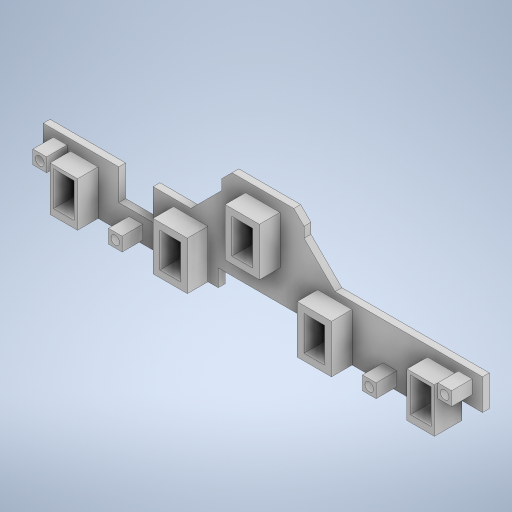
# Autodesk Inventor part: Infravermelhos_revisto_2
Saved by Autodesk Inventor 2024 (Build 280153000, 153)
## iProperties
Created: 2023-04-03
Part Number: Infravermelhos_revisto_2
Material: Generic
Document SubType Name: Modeling
Designer: guilh
Density: 1 g/cm^3
Appearance: Default
Author: guilh
Autodesk Inventor part; units mm, degrees
ref_plane "YZ Plane" through (0, 0, 0) normal (1, 0, 0) x (0, 1, 0)
ref_plane "XZ Plane" through (0, 0, 0) normal (0, 1, 0) x (-1, 0, 0)
ref_plane "XY Plane" through (0, 0, 0) normal (0, 0, 1) x (1, 0, 0)
sketch "Sketch1" plane through (0, 0, 0) normal (0, 0, 1) x (1, 0, 0)
  line L0 (-64, 31) -> (-73, 31)
  line L1 (-76, 28) -> (-76, 25)
  line L2 (-85, 16) -> (-76, 25)
  line L3 (-76, 28) -> (-73, 31)
  line L4 (-64, 31) -> (-55, 31)
  line L5 (-52, 28) -> (-52, 25)
  line L6 (-43, 16) -> (-52, 25)
  line L7 (-52, 28) -> (-55, 31)
  line L8 (-43, 16) -> (0, 16)
  line L9 (-77, 0) -> (-77, 5)
  line L10 (-77, 5) -> (-51, 5)
  line L11 (-51, 5) -> (-51, 0)
  line L12 (-106, 16) -> (-106, 7)
  line L13 (-106, 7) -> (-96, 7)
  line L14 (-96, 7) -> (-96, 16)
  line L15 (-128, 16) -> (-106, 16)
  line L16 (-96, 16) -> (-85, 16)
  line L17 (-120, 0) -> (-120, 7)
  line L18 (-120, 7) -> (-128, 7)
  line L19 (-120, 0) -> (-77, 0)
  line L20 (-128, 16) -> (-128, 7)
  line L21 (-8, 0) -> (-8, 7)
  line L22 (-8, 7) -> (0, 7)
  line L23 (-51, 0) -> (-8, 0)
  line L24 (0, 7) -> (0, 16)
  point P0 (0, 0)
  dimension "d0" = 128
  dimension "d6" = 3
  dimension "d67" = 5
  dimension "d71" = 22
  dimension "d74" = 9
  dimension "d75" = 10
  dimension "d93" = 7
  dimension "d94" = 8
  dimension "d95" = 7
  constraints: 50 end point, 6 horizontal, 3 perpendicular, 2 vertical
  measures "d0" distance of L15.start L8.end
  measures "d6" distance of L1.start L1.end
  measures "d67" distance of L9.start L9.end
  measures "d71" distance of L15.start L12.start
  measures "d74" distance of L12.start L12.end
  measures "d75" distance of L12.end L13.end
  measures "d93" distance of L17.start L17.end
  measures "d94" distance of point (0, 0) L21.start
  measures "d95" distance of L21.start L21.end
extrude "Extrusion1" add sketch "Sketch1" against normal blind 2
sketch "Sketch2" plane through (0, 0, 0) normal (0, 0, 1) x (1, 0, 0)
  line L0 (-119, 2) -> (-113, 2)
  line L1 (-113, 2) -> (-113, 12)
  line L2 (-113, 12) -> (-119, 12)
  line L3 (-119, 12) -> (-119, 2)
  line L4 (-121, 10) -> (-125, 10)
  line L5 (-125, 10) -> (-125, 14)
  line L6 (-125, 14) -> (-121, 14)
  line L7 (-121, 14) -> (-121, 10)
  line L8 (-88, 2) -> (-82, 2)
  line L9 (-82, 2) -> (-82, 12)
  line L10 (-82, 12) -> (-88, 12)
  line L11 (-88, 12) -> (-88, 2)
  line L12 (-90, 0) -> (-80, 0)
  line L13 (-80, 0) -> (-80, 14)
  line L14 (-80, 14) -> (-90, 14)
  line L15 (-90, 14) -> (-90, 0)
  line L16 (-99, 1) -> (-103, 1)
  line L17 (-103, 1) -> (-103, 5)
  line L18 (-103, 5) -> (-99, 5)
  line L19 (-99, 5) -> (-99, 1)
  line L20 (-61, 26) -> (-67, 26)
  line L21 (-67, 26) -> (-67, 16)
  line L22 (-67, 16) -> (-61, 16)
  line L23 (-61, 16) -> (-61, 26)
  line L24 (-59, 14) -> (-69, 14)
  line L25 (-69, 14) -> (-69, 28)
  line L26 (-69, 28) -> (-59, 28)
  line L27 (-59, 28) -> (-59, 14)
  line L28 (-9, 2) -> (-15, 2)
  line L29 (-15, 2) -> (-15, 12)
  line L30 (-15, 12) -> (-9, 12)
  line L31 (-9, 12) -> (-9, 2)
  line L32 (-7, 10) -> (-3, 10)
  line L33 (-3, 10) -> (-3, 14)
  line L34 (-3, 14) -> (-7, 14)
  line L35 (-7, 14) -> (-7, 10)
  line L36 (-40, 2) -> (-46, 2)
  line L37 (-46, 2) -> (-46, 12)
  line L38 (-46, 12) -> (-40, 12)
  line L39 (-40, 12) -> (-40, 2)
  line L40 (-38, 0) -> (-48, 0)
  line L41 (-48, 0) -> (-48, 14)
  line L42 (-48, 14) -> (-38, 14)
  line L43 (-38, 14) -> (-38, 0)
  line L44 (-29, 1) -> (-25, 1)
  line L45 (-25, 1) -> (-25, 5)
  line L46 (-25, 5) -> (-29, 5)
  line L47 (-29, 5) -> (-29, 1)
  line L48 (-112, 13) -> (-120, 13)
  line L49 (-8, 13) -> (-16, 13)
  line L50 (-120, 13) -> (-120, 0)
  line L51 (-112, 13) -> (-112, 0)
  line L52 (-16, 13) -> (-16, 0)
  line L53 (-8, 13) -> (-8, 0)
  circle A0 centre (-123, 12) radius 1.25
  circle A1 centre (-101, 3) radius 1.25
  circle A2 centre (-27, 3) radius 1.25
  circle A3 centre (-5, 12) radius 1.25
  line L54 (-120, 0) -> (-112, 0)
  line L55 (-16, 0) -> (-8, 0)
  dimension "d12" = 6
  dimension "d13" = 10
  dimension "d21" = 6
  dimension "d22" = 10
  dimension "d23" = 2
  dimension "d29" = 6
  dimension "d30" = 10
  dimension "d31" = 2
  dimension "d48" = 1
  dimension "d49" = 2.5
  dimension "d50" = 2.5
  dimension "d51" = 2.5
  dimension "d52" = 2.5
  dimension "d69" = 13
  constraints: 112 end point, 14 parallel, 7 perpendicular, 6 horizontal, 4 centre point, 1 vertical, 6 other
  measures "d12" distance of L2.end L1.end
  measures "d13" distance of L1.end L0.end
  measures "d21" distance of L10.end L9.end
  measures "d22" distance of L9.end L8.end
  measures "d23" distance between parallel lines of L11 L15
  measures "d29" distance of L22.end L21.end
  measures "d30" distance of L21.end L20.end
  measures "d31" distance between parallel lines of L22 L24
  measures "d48" distance between parallel lines of L30 L49
  measures "d49" diameter of A0
  measures "d50" diameter of A1
  measures "d51" diameter of A2
  measures "d52" diameter of A3
  measures "d69" distance of L51.end L48.start
sketch "Sketch10" plane through (0, 0, 0) normal (0, 0, 1) x (1, 0, 0)
  line L0 (-119, 2) -> (-113, 2)
  line L1 (-113, 2) -> (-113, 12)
  line L2 (-113, 12) -> (-119, 12)
  line L3 (-119, 12) -> (-119, 2)
  line L4 (-121, 10) -> (-125, 10)
  line L5 (-125, 10) -> (-125, 14)
  line L6 (-125, 14) -> (-121, 14)
  line L7 (-121, 14) -> (-121, 10)
  line L8 (-88, 2) -> (-82, 2)
  line L9 (-82, 2) -> (-82, 12)
  line L10 (-82, 12) -> (-88, 12)
  line L11 (-88, 12) -> (-88, 2)
  line L12 (-90, 0) -> (-80, 0)
  line L13 (-80, 0) -> (-80, 14)
  line L14 (-80, 14) -> (-90, 14)
  line L15 (-90, 14) -> (-90, 0)
  line L16 (-99, 1) -> (-103, 1)
  line L17 (-103, 1) -> (-103, 5)
  line L18 (-103, 5) -> (-99, 5)
  line L19 (-99, 5) -> (-99, 1)
  line L20 (-61, 26) -> (-67, 26)
  line L21 (-67, 26) -> (-67, 16)
  line L22 (-67, 16) -> (-61, 16)
  line L23 (-61, 16) -> (-61, 26)
  line L24 (-59, 14) -> (-69, 14)
  line L25 (-69, 14) -> (-69, 28)
  line L26 (-69, 28) -> (-59, 28)
  line L27 (-59, 28) -> (-59, 14)
  line L28 (-25, 1) -> (-25, 5)
  line L29 (-9, 2) -> (-15, 2)
  line L30 (-15, 2) -> (-15, 12)
  line L31 (-15, 12) -> (-9, 12)
  line L32 (-9, 12) -> (-9, 2)
  line L33 (-7, 14) -> (-7, 10)
  line L34 (-7, 10) -> (-3, 10)
  line L35 (-3, 10) -> (-3, 14)
  line L36 (-3, 14) -> (-7, 14)
  line L37 (-29, 1) -> (-25, 1)
  line L38 (-25, 5) -> (-29, 5)
  line L39 (-29, 5) -> (-29, 1)
  line L40 (-38, 14) -> (-38, 0)
  line L41 (-40, 12) -> (-40, 2)
  line L42 (-40, 2) -> (-46, 2)
  line L43 (-46, 12) -> (-40, 12)
  line L44 (-46, 2) -> (-46, 12)
  line L45 (-48, 14) -> (-38, 14)
  line L46 (-48, 0) -> (-48, 14)
  line L47 (-38, 0) -> (-48, 0)
  line L48 (-112, 13) -> (-120, 13)
  line L49 (-8, 13) -> (-16, 13)
  circle A0 centre (-123, 12) radius 1.25
  circle A1 centre (-101, 3) radius 1.25
  circle A2 centre (-27, 3) radius 1.25
  circle A3 centre (-5, 12) radius 1.25
  line L50 (-120, 13) -> (-120, 0)
  line L51 (-112, 13) -> (-112, 0)
  line L52 (-112, 0) -> (-120, 0)
  line L53 (-16, 13) -> (-16, 0)
  line L54 (-16, 0) -> (-8, 0)
  line L55 (-8, 13) -> (-8, 0)
  point P0 (-100.5385, 17.107)
  point P1 (-110.5385, 3.107)
  point P2 (-100.5385, 3.107)
  point P3 (-141.5385, 3.107)
  point P4 (-131.5385, 3.107)
  point P5 (-183.5385, 3.107)
  point P6 (-173.5385, 3.107)
  point P7 (-214.5385, 3.107)
  point P8 (-204.5385, 3.107)
  point P9 (-214.5385, 17.107)
  point P10 (0, 16)
  point P11 (0, 0)
  dimension "d53" = 6
  dimension "d54" = 10
  dimension "d55" = 6
  dimension "d56" = 10
  dimension "d57" = 2
  dimension "d58" = 6
  dimension "d59" = 10
  dimension "d60" = 2
  dimension "d61" = 1
  dimension "d62" = 2.5
  dimension "d63" = 2.5
  dimension "d64" = 2.5
  dimension "d65" = 2.5
  constraints: 112 end point, 14 parallel, 9 perpendicular, 5 horizontal, 4 centre point, 3 vertical, 6 other
  measures "d53" distance of L2.end L2.start
  measures "d54" distance of L2.start L0.end
  measures "d55" distance of L11.start L9.end
  measures "d56" distance of L9.end L8.end
  measures "d57" distance between parallel lines of L11 L15
  measures "d58" distance of L22.end L21.end
  measures "d59" distance of L21.end L21.start
  measures "d60" distance between parallel lines of L22 L24
  measures "d61" distance between parallel lines of L31 L49
  measures "d62" diameter of A0
  measures "d63" diameter of A1
  measures "d64" diameter of A2
  measures "d65" diameter of A3
extrude "Extrusion2" cut sketch "Sketch2" against normal blind 2 contours L3 L2 L1 L0 | L11 L10 L9 L8 | L23 L22 L21 L20 | L28 L29 L30 L31 | L36 L37 L38 L39 | A0 | A1 | A2 | A3
extrude "Extrusion7" add sketch "Sketch10" along normal blind 6
body "Solid1"
